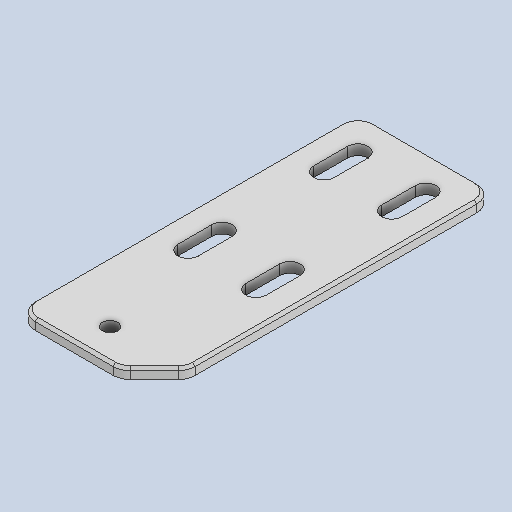
# Autodesk Inventor part: Middle
Saved by Autodesk Inventor 2022 (Build 260153000, 153)
## iProperties
Created: 2021-02-16
Part Number: Middle
Material: Generic
Document SubType Name: Modeling
Designer: Viktor
Density: 1 g/cm^3
Appearance: Default
Author: Viktor
Autodesk Inventor part; units mm, degrees
ref_plane "YZ Plane" through (0, 0, 0) normal (1, 0, 0) x (0, 1, 0)
ref_plane "XZ Plane" through (0, 0, 0) normal (0, 1, 0) x (-1, 0, 0)
ref_plane "XY Plane" through (0, 0, 0) normal (0, 0, 1) x (1, 0, 0)
sketch "Sketch1" plane through (0, 0, 0) normal (0, 1, 0) x (-1, 0, 0)
  line L0 (-20, 50) -> (20, 50)
  line L1 (20, 50) -> (20, -50)
  line L2 (20, -50) -> (-20, -50)
  line L3 (-20, -50) -> (-20, 50)
  line L4 (-20, 50) -> (20, -50) construction
  line L5 (20, 50) -> (-20, -50) construction
  point P0 (0, 0)
  dimension "d0" = 100
  dimension "d1" = 40
  constraints: 12 end point, 2 midpoint, 2 parallel, 1 horizontal, 1 perpendicular
  measures "d0" distance of L0.end L1.end
  measures "d1" distance of L1.end L2.end
extrude "Extrusion1" add sketch "Sketch1" along normal blind 3
sketch "Sketch2" plane through (0, 3, 0) normal (0, 1, 0) x (1, 0, 0)
  line L0 (-10, -10) -> (-10, 0) construction
  line L1 (-7, -10) -> (-7, 0)
  line L2 (-13, 0) -> (-13, -10)
  arc A0 (-13, -10) -> (-7, -10) centre (-10, -10) ccw
  arc A1 (-7, 0) -> (-13, 0) centre (-10, 0) ccw
  line L3 (-32, 15) -> (32, 15) construction
  line L4 (20, 50) -> (-20, 50) projected
  line L5 (0, 82) -> (0, -72) projected
  line L6 (-10, 40) -> (-10, 30) construction
  line L7 (-7, 40) -> (-7, 30)
  line L8 (-13, 30) -> (-13, 40)
  arc A2 (-7, 40) -> (-13, 40) centre (-10, 40) ccw
  arc A3 (-13, 30) -> (-7, 30) centre (-10, 30) ccw
  line L9 (10, -10) -> (10, 0) construction
  line L10 (7, -10) -> (7, 0)
  line L11 (13, 0) -> (13, -10)
  arc A4 (7, -10) -> (13, -10) centre (10, -10) ccw
  arc A5 (13, 0) -> (7, 0) centre (10, 0) ccw
  line L12 (10, 40) -> (10, 30) construction
  line L13 (7, 40) -> (7, 30)
  line L14 (13, 30) -> (13, 40)
  arc A6 (13, 40) -> (7, 40) centre (10, 40) ccw
  arc A7 (7, 30) -> (13, 30) centre (10, 30) ccw
  point P0 (0, 0)
  point P1 (-10, -5)
  point P2 (-10, 35)
  point P3 (10, -5)
  point P4 (10, 35)
  dimension "d4" = 3
  dimension "d5" = 10
  dimension "d6" = 20
  dimension "d7" = 35
  dimension "d8" = 10
  dimension "d24" = 40
  constraints: 34 end point, 21 symmetric about line, 16 point on circle, 8 centre point, 4 tangent, 1 horizontal, 1 midpoint, 1 parallel, 1 vertical, 6 other
  measures "d4" radius of A1
  measures "d5" distance of L2.start L2.end
  measures "d6" distance from line of L3 point (-10, -5)
  measures "d7" distance between parallel lines of L4 L3
  measures "d8" distance from line of L5 point (-10, -5)
  measures "d24" distance of point (-10, 35) point (-10, -5)
sketch "Sketch3" plane through (0, 3, 0) normal (0, 1, 0) x (1, 0, 0)
  circle A0 centre (-2, -41) radius 2.25
  line L0 (-20, -50) -> (20, -50) projected
  line L1 (20, -50) -> (20, 50) projected
  line L2 (-20, 50) -> (-20, -50) projected
  point P0 (0, 0)
  dimension "d9" = 4.5
  dimension "d10" = 9
  dimension "d16" = 18
  constraints: 1 centre point
  measures "d9" diameter of A0
  measures "d10" distance from line of L0 A0.centre
  measures "d16" distance from line of L2 A0.centre
extrude "Extrusion2" cut sketch "Sketch3" against normal blind 3
extrude "Extrusion3" cut sketch "Sketch2" against normal blind 3
chamfer "Chamfer3" distance 10 angle 45 1 edges at (20, 1.5, 50)
fillet "Fillet2" radius 5 5 edges at (20, 1.5, 40) (10, 1.5, 50) (20, 1.5, -50) (-20, 1.5, -50) (-20, 1.5, 50)
chamfer "Chamfer4" distance 0.75 angle 45 10 edges at (20, 3, -3.5355) (18.5355, 3, -48.5355) (0, 3, -50) (-18.5355, 3, -48.5355) (-20, 3, 0) (-18.5355, 3, 48.5355) (-3.5355, 3, 50) (9.8423, 3, 49.6194) (15, 3, 45) (19.6194, 3, 39.8423)
body "Solid1"
